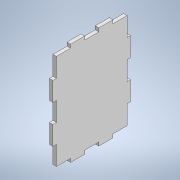
# Autodesk Inventor part: back
Saved by Autodesk Inventor 2020 (Build 240168000, 168)
## iProperties
Created: 2022-02-16
Part Number: back
Material: Generic
Document SubType Name: Modeling
Designer: rwte
Density: 1 g/cm^3
Appearance: Default
Author: rwte
Autodesk Inventor part; units mm, degrees
ref_plane "YZ Plane" through (0, 0, 0) normal (1, 0, 0) x (0, 1, 0)
ref_plane "XZ Plane" through (0, 0, 0) normal (0, 1, 0) x (-1, 0, 0)
ref_plane "XY Plane" through (0, 0, 0) normal (0, 0, 1) x (1, 0, 0)
sketch "Sketch1" plane through (0, 0, 0) normal (1, 0, 0) x (0, 1, 0)
  line L0 (-40.5, 30) -> (-40.5, -30)
  line L1 (-40.5, -30) -> (40.5, -30)
  line L2 (40.5, -30) -> (40.5, 30)
  line L3 (40.5, 30) -> (-40.5, 30)
  line L4 (-40.5, 30) -> (40.5, -30) construction
  line L5 (-40.5, -30) -> (40.5, 30) construction
  line L6 (-40.5, 18) -> (-40.5, 6)
  line L7 (-40.5, 6) -> (-43.5, 6)
  line L8 (-43.5, 6) -> (-43.5, 18)
  line L9 (-43.5, 18) -> (-40.5, 18)
  line L10 (-40.5, -6) -> (-40.5, -18)
  line L11 (-40.5, -18) -> (-43.5, -18)
  line L12 (-43.5, -18) -> (-43.5, -6)
  line L13 (-43.5, -6) -> (-40.5, -6)
  line L14 (-8.1, -30) -> (-8.1, -33)
  line L15 (-8.1, -33) -> (-24.3, -33)
  line L16 (-24.3, -33) -> (-24.3, -30)
  line L17 (-24.3, -30) -> (-8.1, -30)
  line L18 (8.1, -30) -> (24.3, -30)
  line L19 (24.3, -30) -> (24.3, -33)
  line L20 (24.3, -33) -> (8.1, -33)
  line L21 (8.1, -33) -> (8.1, -30)
  line L22 (-60.9, 0) -> (60.9, 0) projected
  line L23 (0, -45.6) -> (0, 42.6) projected
  line L24 (40.5, 18) -> (40.5, 6)
  line L25 (40.5, 6) -> (43.5, 6)
  line L26 (43.5, 6) -> (43.5, 18)
  line L27 (43.5, 18) -> (40.5, 18)
  line L28 (40.5, -6) -> (40.5, -18)
  line L29 (40.5, -18) -> (43.5, -18)
  line L30 (43.5, -18) -> (43.5, -6)
  line L31 (43.5, -6) -> (40.5, -6)
  point P0 (0, 0)
  point P1 (-43.5, -12)
  point P2 (43.5, -12)
  dimension "d0" = 81
  dimension "d1" = 60
  dimension "d2" = 3
  dimension "d3" = 12
  dimension "d4" = 12
  dimension "d5" = 12
  dimension "d6" = 12
  dimension "d7" = 16.2
  dimension "d8" = 16.2
  dimension "d9" = 16.2
  dimension "d10" = 16.2
  constraints: 60 end point, 10 parallel, 9 symmetric about line, 7 perpendicular, 7 point on line, 3 midpoint, 2 vertical, 1 vertical alignment
  measures "d0" distance of L0.end L1.end
  measures "d1" distance of L1.end L2.end
  measures "d2" distance of L8.end L6.start
  measures "d3" vertical distance of L8.end L0.start
  measures "d4" distance of L12.end L7.end
  measures "d5" distance of L7.end L8.end
  measures "d6" distance of L12.end L11.end
  measures "d7" distance of L15.end L14.end
  measures "d8" distance of L19.end L20.end
  measures "d9" distance from line of L0.end L16
  measures "d10" horizontal distance of L1.end L19.end
extrude "Extrusion1" add sketch "Sketch1" along normal blind 3
sketch "Sketch2" plane through (0, 0, 0) normal (-1, 0, 0) x (0, 0, 1)
  line L0 (30, 24.3) -> (30, 8.1) projected
  line L1 (30, 8.1) -> (33, 8.1) projected
  line L2 (33, 24.3) -> (33, 8.1) projected
  line L3 (30, 24.3) -> (33, 24.3) projected
  line L4 (30, -8.1) -> (30, -24.3) projected
  line L5 (30, -24.3) -> (33, -24.3) projected
  line L6 (33, -8.1) -> (33, -24.3) projected
  line L7 (30, -8.1) -> (33, -8.1) projected
  line L8 (30, 24.3) -> (33, 24.3)
  line L9 (33, 24.3) -> (33, 8.1)
  line L10 (33, 8.1) -> (30, 8.1)
  line L11 (30, 8.1) -> (30, 24.3)
  line L12 (30, -8.1) -> (33, -8.1)
  line L13 (33, -8.1) -> (33, -24.3)
  line L14 (33, -24.3) -> (30, -24.3)
  line L15 (30, -24.3) -> (30, -8.1)
  point P0 (0, 0)
  constraints: 16 end point, 4 parallel, 2 horizontal, 2 perpendicular
extrude "Extrusion2" add sketch "Sketch2" against normal blind 3
equation "\"d3\" = 0.2 * d1"
equation "\"d4\" = d3"
equation "\"d5\" = d3"
equation "\"d6\" = d4"
equation "\"d7\" = 0.2 * d0"
equation "\"d8\" = d7"
equation "\"d9\" = d7"
equation "\"d10\" = d8"
equation "\"d11\" = d2"
equation "\"d13\" = d2"
body "Solid1"
